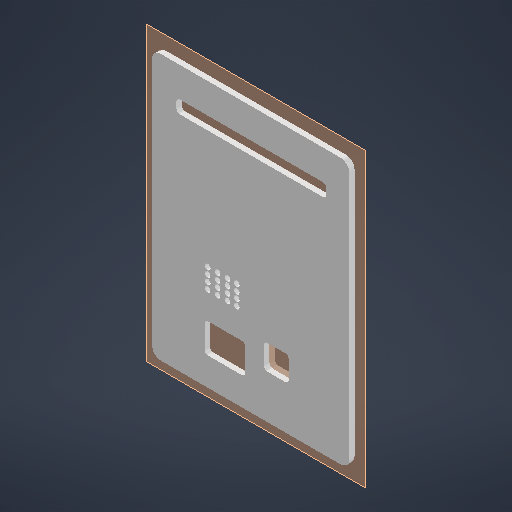
# Autodesk Inventor part: Top
Saved by Autodesk Inventor 2026.3 (Build 303398000, 398)
## iProperties
Created: 2026-09-23
Part Number: Top
Material: Generic
Document SubType Name: Modeling
Designer: arbaz
Density: 1 g/cm^3
Appearance: Default
Author: arbaz
Autodesk Inventor part; units mm, degrees
ref_plane "YZ Plane" through (0, 0, 0) normal (1, 0, 0) x (0, 1, 0)
ref_plane "XZ Plane" through (0, 0, 0) normal (0, 1, 0) x (-1, 0, 0)
ref_plane "XY Plane" through (0, 0, 0) normal (0, 0, 1) x (1, 0, 0)
ref_plane "Work Plane1" through (0, 0, 28.25) normal (0, 0, 1) x (1, 0, 0)
sketch "Sketch2" plane through (0, 0, 28.25) normal (0, 0, 1) x (1, 0, 0)
  line L0 (-30.075, -44.4369) -> (-30.075, -39.9369) projected
  line L1 (-30.075, -39.9369) -> (-25.575, -39.9369) projected
  line L2 (-25.575, -39.9369) -> (-25.575, -44.4369) projected
  line L3 (-25.575, -44.4369) -> (-30.075, -44.4369) projected
  line L4 (31.575, 19.3131) -> (31.575, 14.8131) projected
  line L5 (31.575, 14.8131) -> (27.075, 14.8131) projected
  line L6 (27.075, 14.8131) -> (27.075, 19.3131) projected
  line L7 (27.075, 19.3131) -> (31.575, 19.3131) projected
  line L8 (31.575, -39.9369) -> (31.575, -44.4369) projected
  line L9 (31.575, -44.4369) -> (27.075, -44.4369) projected
  line L10 (27.075, -44.4369) -> (27.075, -39.9369) projected
  line L11 (27.075, -39.9369) -> (31.575, -39.9369) projected
  line L12 (-30.075, 14.8131) -> (-30.075, 19.3131) projected
  line L13 (-30.075, 19.3131) -> (-25.575, 19.3131) projected
  line L14 (-25.575, 19.3131) -> (-25.575, 14.8131) projected
  line L15 (-25.575, 14.8131) -> (-30.075, 14.8131) projected
  line L16 (33.25, -45.75) -> (33.25, 45.75) projected
  line L17 (33.25, 45.75) -> (-33.25, 45.75) projected
  line L18 (-33.25, 45.75) -> (-33.25, -45.75) projected
  line L19 (-33.25, -45.75) -> (33.25, -45.75) projected
  line L20 (-33.25, 45.75) -> (33.25, 45.75)
  line L21 (33.25, 45.75) -> (33.25, -45.75)
  line L22 (33.25, -45.75) -> (-33.25, -45.75)
  line L23 (-33.25, -45.75) -> (-33.25, 45.75)
  line L24 (-33.25, 45.75) -> (33.25, -45.75) construction
  line L25 (33.25, 45.75) -> (-33.25, -45.75) construction
  point P0 (0, 0)
  constraints: 12 end point, 2 midpoint, 2 parallel, 1 horizontal, 1 perpendicular
extrude "Extrusion1" add sketch "Sketch2" against normal blind 1.5 contours L0 L1 L2 L3 | L4 L5 L6 L7 | L8 L9 L10 L11 | L12 L13 L14 L15 | L19 L18 L17 L16
ref_plane "Work Plane2" through (0, 0, 28.25) normal (0, 0, 1) x (1, 0, 0)
sketch "Sketch3" plane through (0, 0, 28.25) normal (0, 0, 1) x (1, 0, 0)
  line L0 (33.25, -45.75) -> (33.25, 45.75) projected
  line L1 (33.25, 45.75) -> (-33.25, 45.75) projected
  line L2 (-33.25, 45.75) -> (-33.25, -45.75) projected
  line L3 (-33.25, -45.75) -> (33.25, -45.75) projected
  line L4 (-33.3375, 49.2125) -> (33.3375, 49.2125)
  line L5 (36.5125, 46.0375) -> (36.5125, -46.0375)
  line L6 (33.3375, -49.2125) -> (-33.3375, -49.2125)
  line L7 (-36.5125, -46.0375) -> (-36.5125, 46.0375)
  line L8 (-36.5125, 49.2125) -> (36.5125, -49.2125) construction
  line L9 (36.5125, 49.2125) -> (-36.5125, -49.2125) construction
  arc A0 (-33.3375, 49.2125) -> (-36.5125, 46.0375) centre (-33.3375, 46.0375) ccw
  arc A1 (-36.5125, -46.0375) -> (-33.3375, -49.2125) centre (-33.3375, -46.0375) ccw
  arc A2 (33.3375, -49.2125) -> (36.5125, -46.0375) centre (33.3375, -46.0375) ccw
  arc A3 (36.5125, 46.0375) -> (33.3375, 49.2125) centre (33.3375, 46.0375) ccw
  point P0 (0, 0)
  dimension "d2" = 3.175
  constraints: 12 end point, 8 point on circle, 8 point on line, 8 tangent, 4 centre point, 3 equal radius, 2 midpoint, 2 parallel, 1 horizontal, 1 perpendicular
  measures "d2" radius of A0
extrude "Extrusion2" add sketch "Sketch3" along normal blind 2 contours L3 L2 L1 L0 | L4 A3 L5 A2 L6 A1 L7 A0
sketch "Sketch4" plane through (0, 0, 26.75) normal (0, 0, -1) x (-1, 0, 0)
  line L0 (-30.1625, 42.8625) -> (30.1625, 42.8625)
  line L1 (30.1625, 42.8625) -> (30.1625, -42.8625)
  line L2 (30.1625, -42.8625) -> (-30.1625, -42.8625)
  line L3 (-30.1625, -42.8625) -> (-30.1625, 42.8625)
  line L4 (-30.1625, 42.8625) -> (30.1625, -42.8625) construction
  line L5 (30.1625, 42.8625) -> (-30.1625, -42.8625) construction
  point P0 (0, 0)
  constraints: 12 end point, 2 midpoint, 2 parallel, 1 horizontal, 1 perpendicular
extrude "Extrusion3" cut sketch "Sketch4" against normal blind 1.5
sketch "Sketch5" plane through (0, 0, 28.25) normal (0, 0, -1) x (-1, 0, 0)
  line L0 (3.175, -42.8625) -> (-21.325, -42.8625)
  line L1 (-21.325, -42.8625) -> (-21.325, -18.3625)
  line L2 (-21.325, -18.3625) -> (3.175, -18.3625)
  line L3 (3.175, -18.3625) -> (3.175, -42.8625)
  point P0 (0, 0)
  dimension "d7" = 24.5
  dimension "d8" = 24.5
  constraints: 8 end point, 2 parallel, 1 horizontal, 1 perpendicular
  measures "d7" distance of L1.end L2.end
  measures "d8" distance of L0.end L1.end
extrude "Extrusion4" add sketch "Sketch5" along normal blind 2
sketch "Sketch6" plane through (0, 0, 26.25) normal (0, 0, -1) x (-1, 0, 0)
  line L0 (-21.325, -42.8625) -> (3.175, -42.8625) projected
  line L1 (-6.17, -23.7643) -> (-12.88, -23.7643)
  line L2 (-14.15, -25.0343) -> (-14.15, -31.7443)
  line L3 (-12.88, -33.0143) -> (-6.17, -33.0143)
  line L4 (-4.9, -31.7443) -> (-4.9, -25.0343)
  line L5 (-4.9, -23.7643) -> (-14.15, -33.0143) construction
  line L6 (-14.15, -23.7643) -> (-4.9, -33.0143) construction
  arc A0 (-14.15, -31.7443) -> (-12.88, -33.0143) centre (-12.88, -31.7443) ccw
  arc A1 (-12.88, -23.7643) -> (-14.15, -25.0343) centre (-12.88, -25.0343) ccw
  arc A2 (-4.9, -25.0343) -> (-6.17, -23.7643) centre (-6.17, -25.0343) ccw
  arc A3 (-6.17, -33.0143) -> (-4.9, -31.7443) centre (-6.17, -31.7443) ccw
  point P0 (0, 0)
  point P1 (-9.525, -28.3893)
  dimension "d13" = 9.25
  dimension "d14" = 9.25
  dimension "d50" = 1.27
  constraints: 12 end point, 8 point on circle, 8 point on line, 8 tangent, 4 centre point, 3 equal radius, 2 midpoint, 2 parallel, 1 horizontal, 1 perpendicular
  measures "d13" distance of L6.end L5.end
  measures "d14" distance of L5.end L6.start
  measures "d50" radius of A0
extrude "Extrusion5" cut sketch "Sketch6" against normal blind 5
sketch "Sketch8" plane through (0, 0, 28.25) normal (0, 0, -1) x (-1, 0, 0)
  line L0 (-21.325, -42.8625) -> (-30.1625, -42.8625) projected
  line L1 (15.755, -38.8375) -> (3.295, -38.8375)
  line L2 (2.025, -37.5675) -> (2.025, -29.1075)
  line L3 (3.295, -27.8375) -> (15.755, -27.8375)
  line L4 (17.025, -29.1075) -> (17.025, -37.5675)
  line L5 (17.025, -38.8375) -> (2.025, -27.8375) construction
  line L6 (2.025, -38.8375) -> (17.025, -27.8375) construction
  arc A0 (2.025, -37.5675) -> (3.295, -38.8375) centre (3.295, -37.5675) ccw
  arc A1 (3.295, -27.8375) -> (2.025, -29.1075) centre (3.295, -29.1075) ccw
  arc A2 (17.025, -29.1075) -> (15.755, -27.8375) centre (15.755, -29.1075) ccw
  arc A3 (15.755, -38.8375) -> (17.025, -37.5675) centre (15.755, -37.5675) ccw
  point P0 (0, 0)
  point P1 (9.525, -33.3375)
  dimension "d20" = 15
  dimension "d21" = 11
  dimension "d51" = 1.27
  constraints: 12 end point, 8 point on circle, 8 point on line, 8 tangent, 4 centre point, 3 equal radius, 2 midpoint, 2 parallel, 1 horizontal, 1 perpendicular
  measures "d20" distance of L5.end L6.end
  measures "d21" distance of L6.start L5.end
  measures "d51" radius of A0
extrude "Extrusion6" cut sketch "Sketch8" against normal blind 5
sketch "Sketch9" plane through (0, 0, 28.25) normal (0, 0, -1) x (-1, 0, 0)
  line L0 (3.295, -27.8375) -> (15.755, -27.8375) projected
  circle A0 centre (15.9202, -17.6714) radius 1
  circle A1 centre (12.2262, -17.6714) radius 1
  circle A2 centre (8.582, -17.6714) radius 1
  circle A3 centre (5.1532, -17.6714) radius 1
  circle A4 centre (15.9202, -15.2556) radius 1
  circle A5 centre (12.2262, -15.2556) radius 1
  circle A6 centre (8.582, -15.2556) radius 1
  circle A7 centre (5.1532, -15.2556) radius 1
  circle A8 centre (15.9202, -12.9089) radius 1
  circle A9 centre (12.2262, -12.9089) radius 1
  circle A10 centre (8.582, -12.9089) radius 1
  circle A11 centre (5.1532, -12.9089) radius 1
  circle A12 centre (15.9202, -10.4834) radius 1
  circle A13 centre (12.2262, -10.4834) radius 1
  circle A14 centre (8.582, -10.4834) radius 1
  circle A15 centre (5.1532, -10.4834) radius 1
  point P0 (0, 0)
  point P1 (17.025, -27.8375)
  point P2 (3.175, -27.8375)
  dimension "d25" = 2
  dimension "d33" = 2
  dimension "d34" = 2
  dimension "d35" = 2
  dimension "d36" = 2
  dimension "d37" = 2
  dimension "d38" = 2
  dimension "d39" = 2
  dimension "d40" = 2
  dimension "d41" = 2
  dimension "d42" = 2
  dimension "d43" = 2
  dimension "d44" = 2
  dimension "d45" = 2
  dimension "d46" = 2
  dimension "d47" = 2
  constraints: 16 centre point
  measures "d25" diameter of A0
  measures "d33" diameter of A1
  measures "d34" diameter of A2
  measures "d35" diameter of A3
  measures "d36" diameter of A4
  measures "d37" diameter of A5
  measures "d38" diameter of A6
  measures "d39" diameter of A7
  measures "d40" diameter of A8
  measures "d41" diameter of A9
  measures "d42" diameter of A10
  measures "d43" diameter of A11
  measures "d44" diameter of A12
  measures "d45" diameter of A13
  measures "d46" diameter of A14
  measures "d47" diameter of A15
extrude "Extrusion7" cut sketch "Sketch9" against normal blind 5 contours A0
sketch "Sketch10" plane through (0, 0, 30.25) normal (0, 0, 1) x (1, 0, 0)
  line L0 (26.7669, 33.3375) -> (-26.2556, 33.3375)
  line L1 (-27.5256, 34.6075) -> (-27.5256, 36.83)
  line L2 (-26.2556, 38.1) -> (26.7669, 38.1)
  line L3 (28.0369, 36.83) -> (28.0369, 34.6075)
  arc A0 (26.7669, 33.3375) -> (28.0369, 34.6075) centre (26.7669, 34.6075) ccw
  arc A1 (28.0369, 36.83) -> (26.7669, 38.1) centre (26.7669, 36.83) ccw
  arc A2 (-27.5256, 34.6075) -> (-26.2556, 33.3375) centre (-26.2556, 34.6075) ccw
  arc A3 (-26.2556, 38.1) -> (-27.5256, 36.83) centre (-26.2556, 36.83) ccw
  point P0 (0, 0)
  dimension "d28" = 1.27
  constraints: 8 end point, 8 point on circle, 8 tangent, 4 centre point, 3 equal radius, 2 parallel, 1 horizontal, 1 perpendicular
  measures "d28" radius of A0
extrude "Extrusion8" cut sketch "Sketch10" against normal blind 5
sketch "Sketch11" plane through (0, 0, 26.25) normal (0, 0, -1) x (-1, 0, 0)
  line L0 (-3.175, -42.8625) -> (-15.875, -42.8625)
  line L1 (-15.875, -42.8625) -> (-15.875, -36.5125)
  line L2 (-15.875, -36.5125) -> (-3.175, -36.5125)
  line L3 (-3.175, -36.5125) -> (-3.175, -42.8625)
  point P0 (0, 0)
  constraints: 8 end point, 2 parallel, 1 horizontal, 1 perpendicular
extrude "Extrusion9" cut sketch "Sketch9" against normal blind 2
fillet "Fillet1" radius 0.127 16 edges at (-4.1532, -17.6714, 30.25) (-7.582, -17.6714, 30.25) (-11.2262, -17.6714, 30.25) (-14.9202, -17.6714, 30.25) (-14.9202, -15.2556, 30.25) (-11.2262, -15.2556, 30.25) (-7.582, -15.2556, 30.25) (-4.1532, -15.2556, 30.25) (-4.1532, -12.9089, 30.25) (-4.1532, -10.4834, 30.25) (-7.582, -10.4834, 30.25) (-7.582, -12.9089, 30.25) (-11.2262, -12.9089, 30.25) (-11.2262, -10.4834, 30.25) (-14.9202, -10.4834, 30.25) (-14.9202, -12.9089, 30.25)
equation "\"d48\" = d25"
body "Solid1"
